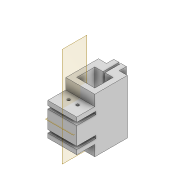
# Autodesk Inventor part: Drone_mount
Saved by Autodesk Inventor 2022 (Build 260153000, 153)
## iProperties
Created: 2022-06-29
Part Number: Drone_mount
Material: Generic
Document SubType Name: Modeling
Designer: dell
Density: 1 g/cm^3
Appearance: Default
Mass: 30.3471 g
Surface Area: 119.338 cm^2
Volume: 30.3471 cm^3
Author: dell
Autodesk Inventor part; units mm, degrees
ref_plane "YZ Plane" through (0, 0, 0) normal (1, 0, 0) x (0, 1, 0)
ref_plane "XZ Plane" through (0, 0, 0) normal (0, 1, 0) x (-1, 0, 0)
ref_plane "XY Plane" through (0, 0, 0) normal (0, 0, 1) x (1, 0, 0)
sketch "Sketch1" plane through (0, 0, 0) normal (0, 0, 1) x (1, 0, 0)
  line L0 (0, 0) -> (32, 0)
  line L1 (32, 0) -> (32, 60)
  line L2 (32, 60) -> (0, 60)
  line L3 (0, 60) -> (0, 0)
  dimension "d0" = 32
  dimension "d1" = 60
  constraints: 8 end point, 2 parallel, 1 horizontal, 1 perpendicular
  measures "d0" distance between parallel lines of L3 L1
  measures "d1" distance between parallel lines of L0 L2
extrude "Extrusion1" add sketch "Sketch1" along normal blind 6
sketch "Sketch3" plane through (0, 0, 6) normal (0, 0, 1) x (1, 0, 0)
  line L0 (32, 0) -> (32, 60) projected
  line L1 (32, 60) -> (0, 60) projected
  line L2 (0, 60) -> (0, 0) projected
  line L3 (0, 0) -> (32, 0) projected
  line L4 (0, 30) -> (32, 30) construction
  line L5 (32, 0) -> (32, 60) construction
  line L6 (0, 60) -> (0, 0) projected
  line L7 (0, 39.9) -> (32, 39.9)
  line L8 (32, 39.9) -> (32, 20.1)
  line L9 (32, 20.1) -> (0, 20.1)
  line L10 (0, 20.1) -> (0, 39.9)
  line L11 (0, 43.1) -> (32, 43.1)
  line L12 (32, 43.1) -> (32, 48.1)
  line L13 (32, 48.1) -> (0, 48.1)
  line L14 (0, 48.1) -> (0, 43.1)
  line L15 (0, 16.9) -> (32, 16.9)
  line L16 (32, 16.9) -> (32, 11.9)
  line L17 (32, 11.9) -> (0, 11.9)
  line L18 (0, 11.9) -> (0, 16.9)
  point P0 (0, 11.9)
  point P1 (0, 20.1)
  point P2 (0, 48.1)
  point P3 (0, 43.1)
  dimension "d6" = 30
  dimension "d7" = 60
  dimension "d8" = 9.9
  dimension "d9" = 9.9
  dimension "d10" = 5
  dimension "d11" = 3.2
  dimension "d12" = 3.2
  dimension "d13" = 5
  constraints: 26 end point, 6 parallel, 6 point on line, 4 perpendicular, 3 horizontal, 2 midpoint
  measures "d6" distance between parallel lines of L3 L4
  measures "d7" distance between parallel lines of L1 L3
  measures "d8" distance between parallel lines of L4 L9
  measures "d9" distance between parallel lines of L4 L7
  measures "d10" distance between parallel lines of L13 L11
  measures "d11" distance between parallel lines of L7 L11
  measures "d12" distance between parallel lines of L9 L15
  measures "d13" distance between parallel lines of L17 L15
extrude "Extrusion2" add sketch "Sketch3" along normal blind 20 contours L17 L2 L15 L0 | L9 L2 L7 L0 | L11 L2 L13 L0
sketch "Sketch4" plane through (0, 48.1, 6) normal (0, 1, 0) x (1, 0, 0)
  line L0 (0, 0) -> (32, 0) projected
  line L1 (0, 0) -> (0, -20) projected
  line L2 (32, -20) -> (0, -20) projected
  line L3 (32, 0) -> (32, -20) projected
  circle A0 centre (11.05, -8) radius 1.55
  circle A1 centre (20.95, -8) radius 1.55
  line L4 (0, -20) -> (32, -20) construction
  line L5 (16, -20) -> (16, 0) construction
  point P0 (0, 6)
  dimension "d16" = 3.1
  dimension "d17" = 3.1
  dimension "d18" = 4.95
  dimension "d19" = 4.95
  dimension "d20" = 8
  dimension "d21" = 8
  constraints: 2 centre point, 2 end point, 2 midpoint
  measures "d16" diameter of A0
  measures "d17" diameter of A1
  measures "d18" distance from line of L5 A0.centre
  measures "d19" distance from line of A1.centre L5
  measures "d20" distance from line of L0 A1.centre
  measures "d21" distance from line of L0 A0.centre
extrude "Extrusion3" cut sketch "Sketch4" against normal blind 100 contours A0 | A1
ref_plane "Work Plane1" through (16, 0, 0) normal (1, 0, 0) x (0, 0, -1)
ref_plane "Work Plane3" through (0, 30, 6) normal (0, 1, 0) x (1, 0, 0)
sketch "Sketch14" plane through (0, 60, 0) normal (0, 1, 0) x (1, 0, 0)
  line L0 (32, 0) -> (0, 0) projected
  line L1 (5.9, 0) -> (26.1, 0)
  line L2 (26.1, 0) -> (26.1, 20.2)
  line L3 (26.1, 20.2) -> (5.9, 20.2)
  line L4 (5.9, 20.2) -> (5.9, 0)
  line L5 (0, 0) -> (32, 0)
  line L6 (32, 0) -> (32, 30)
  line L7 (32, 30) -> (0, 30)
  line L8 (0, 30) -> (0, 0)
  line L9 (32, 0) -> (32, -6) projected
  line L10 (9, 20.2) -> (15, 20.2)
  line L11 (15, 20.2) -> (15, 38)
  line L12 (15, 38) -> (9, 38)
  line L13 (9, 38) -> (9, 20.2)
  line L14 (23, 20.2) -> (17, 20.2)
  line L15 (17, 20.2) -> (17, 38)
  line L16 (17, 38) -> (23, 38)
  line L17 (23, 38) -> (23, 20.2)
  line L18 (16, 46) -> (16, -38) projected
  point P0 (23, 30)
  point P1 (9, 30)
  dimension "d74" = 20.2
  dimension "d75" = 20.2
  dimension "d76" = 30
  dimension "d77" = 5.9
  dimension "d78" = 32
  dimension "d79" = 1
  dimension "d80" = 1
  dimension "d81" = 6
  dimension "d82" = 6
  dimension "d83" = 8
  dimension "d85" = 8
  constraints: 32 end point, 8 parallel, 4 horizontal, 4 perpendicular, 3 point on line, 1 collinear
  measures "d74" distance of L2.end L3.end
  measures "d75" distance of L1.end L2.end
  measures "d76" distance between parallel lines of L0 L7
  measures "d77" distance between parallel lines of L8 L4
  measures "d78" distance of L6.end L7.end
  measures "d79" distance between parallel lines of L18 L15
  measures "d80" distance between parallel lines of L18 L11
  measures "d81" distance between parallel lines of L11 L13
  measures "d82" distance between parallel lines of L15 L17
  measures "d83" distance between parallel lines of L7 L16
  measures "d85" distance between parallel lines of L12 L7
extrude "Extrusion12" add sketch "Sketch14" against normal blind 60 contours L0 L2 L3 L17 L7 L6 | L17 L3 L15 L7 | L7 L15 L16 L17 | L0 L8 L7 L13 L3 L4 | L3 L13 L7 L11 | L7 L13 L12 L11
sketch "Sketch15" plane through (23, 60, -30) normal (1, 0, 0) x (0, 0, -1)
  circle A0 centre (4, -10) radius 1.6
  circle A1 centre (4, -30) radius 1.6
  circle A2 centre (4, -50) radius 1.6
  line L0 (8, -60) -> (0, -60) projected
  line L1 (0, 0) -> (8, 0) projected
  line L2 (8, 0) -> (8, -60) projected
  point P0 (-30, -60)
  dimension "d88" = 3.2
  dimension "d89" = 3.2
  dimension "d90" = 3.2
  dimension "d91" = 10
  dimension "d92" = 10
  dimension "d93" = 30
  dimension "d94" = 4
  constraints: 3 centre point, 2 vertical alignment
  measures "d88" diameter of A0
  measures "d89" diameter of A1
  measures "d90" diameter of A2
  measures "d91" distance from line of L0 A2.centre
  measures "d92" distance from line of A0.centre L1
  measures "d93" distance from line of L0 A1.centre
  measures "d94" distance from line of L2 A0.centre
extrude "Extrusion13" cut sketch "Sketch15" against normal blind 60
sketch "Sketch16" plane through (0, 0, 6) normal (0, 0, 1) x (1, 0, 0)
  line L0 (0, 39.9) -> (32, 39.9) projected
  line L1 (32, 39.9) -> (32, 43.1) projected
  line L2 (32, 43.1) -> (0, 43.1) projected
  line L3 (0, 43.1) -> (0, 39.9) projected
  line L4 (0, 16.9) -> (32, 16.9) projected
  line L5 (32, 16.9) -> (32, 20.1) projected
  line L6 (32, 20.1) -> (0, 20.1) projected
  line L7 (0, 20.1) -> (0, 16.9) projected
  point P0 (0, 0)
extrude "Extrusion14" cut sketch "Sketch16" against normal blind 1
equation "\"d6\" = 0.5 * d7"
equation "\"d77\" = -0.5 * d74 + 0.5 * d78"
body "Solid1"
